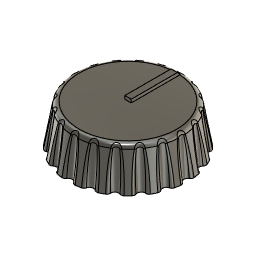
Assembley (Autodesk Fusion 360 archive; units mm, degrees)
design "Knob1"
Autodesk Fusion 360 part; units mm, degrees
sketch "Sketch1" plane through (0, 0, 0) normal (1, 0, 0) x (0, 1, 0)
  line L0 (0, 0) -> (0, -1.5875)
  line L1 (0, -1.5875) -> (1.5875, -1.5875)
  line L2 (1.5875, -1.5875) -> (1.5875, 0)
  line L3 (1.5875, 0) -> (9.525, 0)
  line L4 (9.525, 0) -> (8.4053, 6.35)
  line L5 (8.4053, 6.35) -> (0, 6.35)
  line L6 (0, 6.35) -> (0, 0)
  dimension "d1" = 3.175
  dimension "d2" = 19.05
  dimension "d3" = 6.35
  dimension "d4" = 80
  dimension "d5" = 1.5875
  constraint coincident L0.start L6.end
  constraint vertical L0
  constraint perpendicular L0 L1
  constraint perpendicular L1 L2
  constraint perpendicular L2 L3
  constraint perpendicular L2 L5
  constraint vertical L6
  constraint coincident L0.start L3
  measures "d3" distance of L5.end L0.start
  measures "d4" angle of L3 L4
  measures "d5" distance of L1.end L2.end
revolve "Revolve1" add sketch "Sketch1" angle 360 about axis through (0, 0, 6.35) along (0, 0, -1)
sketch "Sketch2" plane through (0, 0, 0) normal (0, 0, -1) x (1, 0, 0)
  circle A0 centre (0, 0) radius 9.525
  circle A1 centre (0, 0) radius 1.5875
  circle A2 centre (0, 9.525) radius 0.635
  dimension "d7" = 1.27
  constraint coincident A0 A2.centre
  constraint vertical A0.centre A2.centre
  measures "d7" diameter of A2
fillet "Fillet1" radius 0.762 1 edges at (-7.8365, 3.0395, 6.35)
extrude "Extrude1" cut sketch "Sketch2" against normal blind 6.35 draft 5 contours A0 A2 | A0 A2 picked at (0.0155, 9.3123) picked at (-0.0035, 9.7351)
fillet "Fillet2" radius 0.508 3 edges at (-0.7077, -8.9952, 2.8472) (0.0003, -8.3593, 6.0661) (0.7077, -8.9952, 2.8472)
pattern_circular "C-Pattern1" count 20 over 360 about axis through (0, 0, 1.75) along (0, 0, 1) of "Extrude1", "Fillet2"
sketch "Sketch3" plane through (0, 0, 6.35) normal (0, 0, 1) x (-1, 0, 0)
  circle A0 centre (0, 0) radius 7.7659
  line L0 (-0.508, 0) -> (0.508, 0)
  line L1 (0.508, 0) -> (0.508, -7.7493)
  line L2 (0.508, -7.7493) -> (-0.508, -7.7493)
  line L3 (-0.508, -7.7493) -> (-0.508, 0)
  line L4 (-0.508, 0) -> (0.508, -7.7493) construction
  line L5 (0.508, 0) -> (-0.508, -7.7493) construction
  point P0 (0, -3.8746)
  dimension "d14" = 1.016
  constraint perpendicular L0 L1
  constraint parallel L0 L2
  constraint parallel L1 L3
  constraint horizontal L0
  constraint coincident L4 P0
  constraint coincident L5 P0
  constraint midpoint A0.centre L0
  constraint coincident A0 L2.end
  measures "d14" distance of L0.start L0.end
extrude "Extrude2" add sketch "Sketch3" along normal blind 0.508 contours A0 L2 | L0 L1 L2 L3
chamfer "Chamfer1" distance 0.3998 angle 45 1 edges at (0, 7.7659, 6.858)
